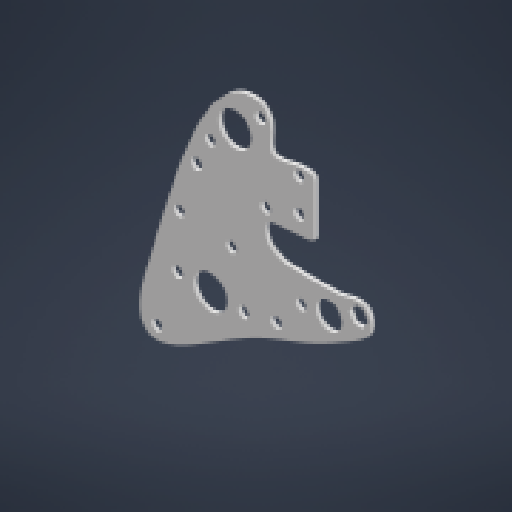
# Autodesk Inventor part: third-stage
Saved by Autodesk Inventor 2023.2 (Build 272271000, 271)
## iProperties
Created: 2023-03-29
Part Number: third-stage
Material: Generic
Document SubType Name: Modeling
Designer: Liam
Density: 1 g/cm^3
Appearance: Default
Author: Liam
Autodesk Inventor part; units mm, degrees
ref_plane "YZ Plane" through (0, 0, 0) normal (1, 0, 0) x (0, 1, 0)
ref_plane "XZ Plane" through (0, 0, 0) normal (0, 1, 0) x (-1, 0, 0)
ref_plane "XY Plane" through (0, 0, 0) normal (0, 0, 1) x (1, 0, 0)
sketch "Sketch1" plane through (0, 0, 0) normal (0, 0, 1) x (1, 0, 0)
  circle A0 centre (-45.6184, 44.45) radius 2.0955
  circle A1 centre (-45.6184, 57.15) radius 2.0955
  circle A2 centre (-79.3648, 1.8096) radius 6.35
  circle A3 centre (-58.2829, 40.2547) radius 2.0955
  circle A4 centre (-84.7892, 41.664) radius 2.0955
  circle A5 centre (-66.6703, 1.4359) radius 2.0955
  circle A6 centre (-92.0593, 2.1834) radius 2.0955
  circle A7 centre (-71.4316, 20.7646) radius 2.0955
  circle A8 centre (-91.4447, 22.7695) radius 2.0955
  circle A9 centre (-69.9964, 60.5103) radius 6.35
  circle A10 centre (-60.4479, 68.8837) radius 2.0955
  circle A11 centre (-79.545, 52.1369) radius 2.0955
  line L0 (-26.356, 22.0475) -> (-24.4745, 18.8943)
  line L1 (-24.4745, 18.8943) -> (-20.8087, 18.9471)
  line L2 (-20.8087, 18.9471) -> (-19.0215, 22.1481)
  line L3 (-19.0215, 22.1481) -> (-20.903, 25.3013)
  line L4 (-20.903, 25.3013) -> (-24.5688, 25.2486)
  line L5 (-24.5688, 25.2486) -> (-26.356, 22.0475)
  line L6 (-39.6875, 58.2598) -> (-39.6875, 39.116)
  circle A12 centre (-54.2866, 4.2789) radius 2.0955
  circle A13 centre (-34.0057, 16.7254) radius 5.08
  line L7 (-39.6875, 39.116) -> (-39.6875, 37.4439) construction
  line L8 (-39.6875, 37.4439) -> (-55.1487, 37.4439) construction
  line L9 (-55.1487, 37.4439) -> (-58.0806, 36.4121) construction
  line L10 (-58.0806, 36.4121) -> (-58.8644, 33.737) construction
  line L11 (-58.8644, 33.737) -> (-57.2052, 24.865) construction
  line L12 (-57.2052, 24.865) -> (-41.919, 25.4146) construction
  line L13 (-41.919, 25.4146) -> (-33.1287, 25.1254) construction
  line L14 (-33.1287, 25.1254) -> (-28.5377, 25.7038) construction
  line L15 (-28.5377, 25.7038) -> (-25.7515, 26.8992) construction
  line L16 (-25.7515, 26.8992) -> (-18.5104, 27.9819) construction
  line L17 (-18.5104, 27.9819) -> (-15.9484, 16.9979) construction
  line L18 (-15.9484, 16.9979) -> (-26.1912, 12.2228) construction
  line L19 (-26.1912, 12.2228) -> (-35.1067, 6.3744) construction
  line L20 (-35.1067, 6.3744) -> (-49.491, 0.0879) construction
  line L21 (-49.491, 0.0879) -> (-66.6703, -4.9887) construction
  line L22 (-66.6703, -4.9887) -> (-102.0203, -32.2212) construction
  line L23 (-102.0203, -32.2212) -> (-109.4018, -17.6163) construction
  line L24 (-109.4018, -17.6163) -> (-102.0203, 2.1834) construction
  line L25 (-102.0203, 2.1834) -> (-95.3545, 27.1384) construction
  line L26 (-95.3545, 27.1384) -> (-88.055, 47.2768) construction
  line L27 (-88.055, 47.2768) -> (-81.0906, 62.0354) construction
  line L28 (-81.0906, 62.0354) -> (-73.0148, 72.0287) construction
  line L29 (-73.0148, 72.0287) -> (-64.5748, 75.7535) construction
  line L30 (-64.5748, 75.7535) -> (-57.0215, 73.4397) construction
  line L31 (-57.0215, 73.4397) -> (-55.8301, 67.032) construction
  line L32 (-55.8301, 67.032) -> (-56.9846, 61.9075) construction
  line L33 (-56.9846, 61.9075) -> (-55.8301, 57.8881) construction
  line L34 (-55.8301, 57.8881) -> (-50.2468, 59.2455) construction
  line L35 (-50.2468, 59.2455) -> (-44.1506, 61.0067) construction
  line L36 (-44.1506, 61.0067) -> (-39.6875, 60.5103) construction
  line L37 (-39.6875, 60.5103) -> (-39.6875, 58.2598) construction
  spline S0 degree 4 poles (-39.6875, 39.116) (-39.6875, 37.4439) (-55.1487, 37.4439) (-58.0806, 36.4121) (-58.8644, 33.737) (-57.2052, 24.865) (-41.919, 25.4146) (-33.1287, 25.1254) (-28.5377, 25.7038) (-25.7515, 26.8992) (-18.5104, 27.9819) (-15.9484, 16.9979) (-26.1912, 12.2228) (-35.1067, 6.3744) (-49.491, 0.0879) (-66.6703, -4.9887) (-102.0203, -32.2212) (-109.4018, -17.6163) (-102.0203, 2.1834) (-95.3545, 27.1384) (-88.055, 47.2768) (-81.0906, 62.0354) (-73.0148, 72.0287) (-64.5748, 75.7535) (-57.0215, 73.4397) (-55.8301, 67.032) (-56.9846, 61.9075) (-55.8301, 57.8881) (-50.2468, 59.2455) (-44.1506, 61.0067) (-39.6875, 60.5103) (-39.6875, 58.2598) knots 1 1 1 1 1 2 3 4 5 6 7 8 9 10 11 12 13 14 15 16 17 18 19 20 21 22 23 24 25 26 27 28 29 29 29 29 29
  circle A14 centre (-44.7526, 14.9681) radius 2.0955
  circle A15 centre (-99.9248, -19.3432) radius 2.0955
  point P0 (0, 0)
  point P1 (-79.3931, 52.0233)
  point P2 (-60.4186, 72.0287)
  point P3 (-81.0906, 53.8995)
  dimension "d23" = 4.191
  dimension "d24" = 4.191
  dimension "d60" = 4.191
  dimension "d61" = 4.191
  dimension "d62" = 12.7
  dimension "d63" = 4.191
  dimension "d64" = 4.191
  dimension "d65" = 12.7
  dimension "d68" = 4.191
  dimension "d69" = 4.191
  dimension "d70" = 12.7
  dimension "d71" = 4.191
  dimension "d72" = 4.191
  dimension "d73" = 4.191
  dimension "d76" = 10.16
  dimension "d77" = 4.191
  dimension "d78" = 4.191
  constraints: 16 centre point, 14 end point, 3 parallel, 2 vertical, 1 horizontal, 26 other
  measures "d23" diameter of A0
  measures "d24" diameter of A1
  measures "d60" diameter of A3
  measures "d61" diameter of A4
  measures "d62" diameter of A2
  measures "d63" diameter of A5
  measures "d64" diameter of A6
  measures "d65" distance of A2.centre A6.centre
  measures "d68" diameter of A7
  measures "d69" diameter of A8
  measures "d70" diameter of A9
  measures "d71" diameter of A10
  measures "d72" diameter of A11
  measures "d73" diameter of A12
  measures "d76" diameter of A13
  measures "d77" diameter of A14
  measures "d78" diameter of A15
extrude "Extrusion5" add sketch "Sketch1" along normal blind 1.524
body "Solid5"
